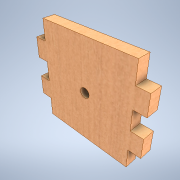
# Autodesk Inventor part: FRONT V2
Saved by Autodesk Inventor 2021.2 (Build 252289000, 289)
## iProperties
Created: 2021-03-11
Part Number: FRONT V2
Material: Wood (Cherry)
Document SubType Name: Modeling
Designer: 443201246
Density: 0.63 g/cm^3
Appearance: Cherry - Natural Low Gloss
Author: 443201246
Autodesk Inventor part; units mm, degrees
ref_plane "YZ Plane" through (0, 0, 0) normal (1, 0, 0) x (0, 1, 0)
ref_plane "XZ Plane" through (0, 0, 0) normal (0, 1, 0) x (-1, 0, 0)
ref_plane "XY Plane" through (0, 0, 0) normal (0, 0, 1) x (1, 0, 0)
sketch "Sketch1" plane through (0, 0, 0) normal (0, 0, 1) x (1, 0, 0)
  line L0 (-59.5, -50) -> (59.5, -50)
  line L1 (59.5, -50) -> (59.5, 50)
  line L2 (59.5, 50) -> (-59.5, 50)
  line L3 (-59.5, 50) -> (-59.5, -50)
  line L4 (-59.5, -50) -> (59.5, 50) construction
  line L5 (59.5, -50) -> (-59.5, 50) construction
  point P0 (0, 0)
  dimension "d0" = 119
  dimension "d1" = 100
  constraints: 12 end point, 2 midpoint, 2 parallel, 1 horizontal, 1 perpendicular
  measures "d0" distance of L2.end L1.end
  measures "d1" distance of L1.end L0.end
extrude "Extrusion1" add sketch "Sketch1" along normal mid plane 12
sketch "Sketch2" plane through (0, 0, 6) normal (0, 0, 1) x (1, 0, 0)
  line L0 (-59.5, 50) -> (-59.5, -50) projected
  line L1 (-59.5, -50) -> (59.5, -50) projected
  line L2 (-59.5, -50) -> (-47.5, -50)
  line L3 (-47.5, -50) -> (-47.5, -30)
  line L4 (-47.5, -30) -> (-59.5, -30)
  line L5 (-59.5, -30) -> (-59.5, -50)
  line L6 (-59.5, -10) -> (-47.5, -10)
  line L7 (-47.5, -10) -> (-47.5, 10)
  line L8 (-47.5, 10) -> (-59.5, 10)
  line L9 (-59.5, 10) -> (-59.5, -10)
  line L10 (-59.5, -50) -> (-59.5, 50) projected
  line L11 (-59.5, 30) -> (-47.5, 30)
  line L12 (-47.5, 30) -> (-47.5, 50)
  line L13 (-47.5, 50) -> (-59.5, 50)
  line L14 (-59.5, 50) -> (-59.5, 30)
  point P0 (0, 0)
  dimension "d17" = 12
  dimension "d18" = 20
  dimension "d19" = 12
  dimension "d20" = 20
  dimension "d21" = 20
  dimension "d22" = 12
  dimension "d23" = 20
  dimension "d24" = 20
  constraints: 24 end point, 6 parallel, 3 horizontal, 3 perpendicular, 2 point on line
  measures "d17" distance of L4.end L3.end
  measures "d18" distance of L3.end L2.end
  measures "d19" distance of L8.end L7.end
  measures "d20" distance of L7.end L6.end
  measures "d21" distance between parallel lines of L4 L6
  measures "d22" distance of L13.end L12.end
  measures "d23" distance of L12.end L11.end
  measures "d24" distance between parallel lines of L11 L8
extrude "Extrusion2" cut sketch "Sketch2" against normal through all
mirror "Mirror1" about plane through (0, 0, 0) normal (1, 0, 0) of "Extrusion2"
sketch "Sketch5" plane through (0, 0, 6) normal (0, 0, 1) x (1, 0, 0)
  circle A0 centre (0, 0) radius 5
  dimension "d25" = 10
  constraints: 1 centre point, 1 coincident
  measures "d25" diameter of A0
extrude "Extrusion4" cut sketch "Sketch5" against normal through all
body "Solid1"
